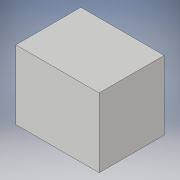
# Autodesk Inventor part: WinchVolume
Saved by Autodesk Inventor 2018.2 (Build 222227000, 227)
## iProperties
Created: 2018-01-31
Part Number: WinchVolume
Material: Generic
Document SubType Name: Modeling
Designer: steele
Density: 1 g/cm^3
Appearance: Default
Author: steele
Autodesk Inventor part; units mm, degrees
ref_plane "YZ Plane" through (0, 0, 0) normal (1, 0, 0) x (0, 1, 0)
ref_plane "XZ Plane" through (0, 0, 0) normal (0, 1, 0) x (-1, 0, 0)
ref_plane "XY Plane" through (0, 0, 0) normal (0, 0, 1) x (1, 0, 0)
sketch "Sketch1" plane through (0, 0, 0) normal (0, 1, 0) x (-1, 0, 0)
  line L0 (65.0875, 50.8) -> (-65.0875, 50.8)
  line L1 (-65.0875, 50.8) -> (-65.0875, -50.8)
  line L2 (-65.0875, -50.8) -> (65.0875, -50.8)
  line L3 (65.0875, -50.8) -> (65.0875, 50.8)
  line L4 (65.0875, 50.8) -> (-65.0875, -50.8) construction
  line L5 (-65.0875, 50.8) -> (65.0875, -50.8) construction
  point P0 (0, 0)
  dimension "d0" = 130.175
  dimension "d1" = 101.6
  constraints: 12 end point, 2 midpoint, 2 parallel, 1 horizontal, 1 perpendicular
  measures "d0" distance of L0.start L0.end
  measures "d1" distance of L1.end L0.end
extrude "Extrusion1" add sketch "Sketch1" along normal blind 107.95
body "Solid1"
